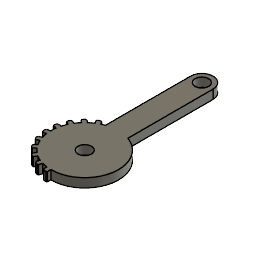
Record 11 3rd part (Autodesk Fusion 360 design; units mm, degrees)
part number: 2026-03-10-15-59-10-716
Autodesk Fusion 360 part; units mm, degrees
sketch "Sketch1" plane through (0, 0, 0) normal (0, 1, 0) x (1, 0, 0)
  circle A0 centre (0.0008, 24.9355) radius 3
  line L0 (2.5556, 32.9383) -> (-2.4444, 32.9383)
  line L1 (2.5556, 20.6375) -> (2.5556, -15.7025)
  line L2 (8, 25) -> (8, -20)
  circle A1 centre (0, -20) radius 3
  line L3 (-2.6799, 20.7149) -> (-2.6799, -15.7789)
  arc A2 (2.5556, 20.6375) -> (-2.6799, 20.7149) centre (0.0008, 24.9355) ccw
  arc A3 (-2.6799, -15.7789) -> (2.5556, -15.7025) centre (0, -20) ccw
  dimension "d1" = 6
  dimension "d2" = 10
  dimension "d4" = 5
  dimension "d5" = 36.34
  dimension "d6" = 45
  dimension "d7" = 6
  constraint concentric A0 A2
  constraint perpendicular L0 L1
  constraint vertical L2
  constraint concentric A1 A3
  constraint vertical L3
  constraint vertical L1
  measures "d1" diameter of A0
  measures "d2" diameter of A2
  measures "d4" distance of L0.start L0.end
  measures "d5" distance of L1.start L1.end
  measures "d6" distance of L2.start L2.end
  measures "d7" diameter of A1
sketch "Sketch2" plane through (0, 0, 0) normal (0, 1, 0) x (1, 0, 0)
  circle A0 centre (160, 0) radius 3
  line L0 (165.3043, -12.1067) -> (165.3043, 17.8933)
  line L1 (165.3043, -12.1067) -> (144.0787, -27.9224)
  line L2 (144.0787, -27.9224) -> (124.0787, -27.9224)
  line L3 (124.0787, -27.9224) -> (105.4535, -9.1138)
  line L4 (105.4535, -9.1138) -> (98.3535, -9.1138)
  line L5 (98.3535, -9.1138) -> (98.3535, 10.8862)
  line L6 (98.3535, 10.8862) -> (112.5535, 10.8862)
  line L7 (112.5535, 10.8862) -> (128, 34)
  line L8 (128, 34) -> (153, 34)
  line L9 (153, 34) -> (165.3043, 17.8933)
  circle A1 centre (144.0787, -15.0238) radius 3
  circle A2 centre (124.0787, -15.0238) radius 3
  line L10 (112.4283, -2.9974) -> (127.553, -3)
  line L11 (127.2855, 2.988) -> (112.556, 3)
  arc A3 (127.553, -3) -> (127.2855, 2.988) centre (127.5535, 0) ccw
  arc A4 (112.556, 3) -> (112.6778, -2.9974) centre (112.5535, 0) ccw
  circle A5 centre (128, 28) radius 2
  circle A6 centre (153, 28) radius 2
  dimension "d10" = 6
  dimension "d11" = 30
  dimension "d12" = 26.47
  dimension "d13" = 20
  dimension "d14" = 26.47
  dimension "d15" = 7.1
  dimension "d16" = 20
  dimension "d17" = 14.2
  dimension "d18" = 27.8
  dimension "d19" = 25
  dimension "d21" = 6
  dimension "d22" = 6
  dimension "d23" = 6
  dimension "d24" = 15
  dimension "d25" = 6
  dimension "d26" = 4
  dimension "d27" = 4
  constraint vertical L0
  constraint horizontal L2
  constraint horizontal L4
  constraint perpendicular L4 L5
  constraint perpendicular L5 L6
  constraint horizontal L8
  constraint coincident L10.start A4
  constraint tangent L10 A3
  constraint tangent L11 A4
  constraint coincident L10 A4.end
  measures "d10" diameter of A0
  measures "d11" distance of L0.start L0.end
  measures "d12" distance of L0.start L1.end
  measures "d13" distance of L1.end L2.end
  measures "d14" distance of L2.end L3.end
  measures "d15" distance of L3.end L4.end
  measures "d16" distance of L4.end L5.end
  measures "d17" distance of L5.end L6.end
  measures "d18" distance of L6.end L7.end
  measures "d19" distance of L7.end L8.end
  measures "d21" diameter of A1
  measures "d22" diameter of A2
  measures "d23" diameter of A4
  measures "d24" distance of A4.centre A3.centre
  measures "d25" diameter of A3
  measures "d26" diameter of A5
  measures "d27" diameter of A6
sketch "Sketch3" plane through (0, 0, 0) normal (0, 1, 0) x (1, 0, 0)
sketch "Sketch4" plane through (0, 0, 0) normal (0, 1, 0) x (1, 0, 0)
sketch "Sketch5" plane through (0, 0, 0) normal (0, 1, 0) x (1, 0, 0)
  circle A0 centre (0, -75) radius 3
  circle A1 centre (-0.0243, -126.973) radius 3
  line L0 (-20, -70) -> (-20, -141.97)
  line L1 (-5, -75) -> (-5, -112.8223)
  line L2 (5, -75) -> (5, -112.8395)
  arc A2 (5, -75) -> (-5, -75) centre (0, -75) ccw
  line L3 (-0.05, -141.973) -> (-0.05, -143.513)
  line L4 (-0.05, -143.513) -> (-0.4621, -143.739)
  line L5 (-0.4621, -143.739) -> (-1.4621, -143.739)
  line L6 (-1.4621, -143.739) -> (-1.9628, -143.2357)
  line L7 (-1.9628, -143.2357) -> (-1.9628, -141.8472)
  line L8 (-0.05, -145.0973) -> (-0.05, -123.9731)
  line L9 (-8.7204, -112.6318) -> (-7.8791, -112.0912)
  line L10 (-8.9448, -113.0448) -> (-8.7204, -112.6318)
  line L11 (-8.1122, -114.3403) -> (-8.9448, -113.0448)
  line L12 (-7.1857, -112.2439) -> (-6.4351, -113.412)
  line L13 (-7.8791, -112.0912) -> (-7.1857, -112.2439)
  line L14 (-12.4085, -115.6627) -> (-11.7536, -114.907)
  line L15 (-12.5075, -116.1222) -> (-12.4085, -115.6627)
  line L16 (-11.3436, -117.1306) -> (-12.5075, -116.1222)
  line L17 (-11.0453, -114.8581) -> (-9.996, -115.7674)
  line L18 (-11.7536, -114.907) -> (-11.0453, -114.8581)
  line L19 (-15.0933, -119.6099) -> (-14.6779, -118.7003)
  line L20 (-15.0589, -120.0786) -> (-15.0933, -119.6099)
  line L21 (-13.658, -120.7184) -> (-15.0589, -120.0786)
  line L22 (-14.012, -118.4539) -> (-12.749, -119.0307)
  line L23 (-14.6779, -118.7003) -> (-14.012, -118.4539)
  line L24 (-16.5573, -124.1536) -> (-16.415, -123.1638)
  line L25 (-16.3922, -124.5936) -> (-16.5573, -124.1536)
  line L26 (-14.8679, -124.8128) -> (-16.3922, -124.5936)
  line L27 (-15.8455, -122.7398) -> (-14.4712, -122.9374)
  line L28 (-16.415, -123.1638) -> (-15.8455, -122.7398)
  line L29 (-16.682, -128.9257) -> (-16.8243, -127.9359)
  line L30 (-16.3995, -129.3014) -> (-16.682, -128.9257)
  line L31 (-14.8752, -129.0822) -> (-16.3995, -129.3014)
  line L32 (-16.3973, -127.3686) -> (-15.023, -127.171)
  line L33 (-16.8243, -127.9359) -> (-16.3973, -127.3686)
  line L34 (-15.4571, -133.5396) -> (-15.8725, -132.63)
  line L35 (-15.0802, -133.8205) -> (-15.4571, -133.5396)
  line L36 (-13.6794, -133.1808) -> (-15.0802, -133.8205)
  line L37 (-15.6226, -131.9654) -> (-14.3596, -131.3886)
  line L38 (-15.8725, -132.63) -> (-15.6226, -131.9654)
  line L39 (-12.9819, -137.6215) -> (-13.6367, -136.8658)
  line L40 (-12.5412, -137.7849) -> (-12.9819, -137.6215)
  line L41 (-11.3773, -136.7764) -> (-12.5412, -137.7849)
  line L42 (-13.5843, -136.1577) -> (-12.5349, -135.2485)
  line L43 (-13.6367, -136.8658) -> (-13.5843, -136.1577)
  line L44 (-9.457, -140.8408) -> (-10.2982, -140.3002)
  line L45 (-8.9881, -140.8734) -> (-9.457, -140.8408)
  line L46 (-8.1555, -139.5779) -> (-8.9881, -140.8734)
  line L47 (-10.4473, -139.606) -> (-9.6967, -138.4379)
  line L48 (-10.2982, -140.3002) -> (-10.4473, -139.606)
  line L49 (-5.1679, -142.9365) -> (-6.1274, -142.6548)
  line L50 (-4.7088, -142.8357) -> (-5.1679, -142.9365)
  line L51 (-4.2749, -141.3581) -> (-4.7088, -142.8357)
  line L52 (-6.466, -142.0308) -> (-6.0748, -140.6985)
  line L53 (-6.1274, -142.6548) -> (-6.466, -142.0308)
  arc A3 (-5, -112.8223) -> (-6.4351, -113.412) centre (-0.0243, -126.973) ccw
  arc A4 (-8.1122, -114.3403) -> (-9.996, -115.7674) centre (-0.0243, -126.973) ccw
  arc A5 (-11.3436, -117.1306) -> (-12.749, -119.0307) centre (-0.0243, -126.973) ccw
  arc A6 (-13.658, -120.7184) -> (-14.4712, -122.9374) centre (-0.0243, -126.973) ccw
  arc A7 (-14.8679, -124.8128) -> (-15.023, -127.171) centre (-0.0243, -126.973) ccw
  arc A8 (-14.8752, -129.0822) -> (-14.3596, -131.3886) centre (-0.0243, -126.973) ccw
  arc A9 (-13.6794, -133.1808) -> (-12.5349, -135.2485) centre (-0.0243, -126.973) ccw
  arc A10 (-11.3773, -136.7764) -> (-9.6967, -138.4379) centre (-0.0243, -126.973) ccw
  arc A11 (-8.1555, -139.5779) -> (-6.0748, -140.6985) centre (-0.0243, -126.973) ccw
  arc A12 (-4.2749, -141.3581) -> (-1.9628, -141.8472) centre (-0.0243, -126.973) ccw
  arc A13 (-0.05, -141.973) -> (5, -112.8395) centre (-0.0243, -126.973) ccw
  dimension "d30" = 6
  dimension "d31" = 10
  dimension "d32" = 6
  dimension "d33" = 30
  dimension "d34" = 71.97
  dimension "d35" = 1.54
  dimension "d36" = 0.47
  dimension "d37" = 1
  dimension "d38" = 0.71
  dimension "d40" = 360
  constraint concentric A0 A2
  constraint concentric A1 A4
  constraint vertical L0
  constraint vertical L1
  constraint tangent L2 A2
  constraint parallel L1 L2
  constraint vertical L3
  constraint horizontal L5
  constraint vertical L7
  constraint vertical L8
  constraint coincident A1 L8.end
  constraint concentric A3 A4
  constraint concentric A4 A5
  constraint concentric A5 A6
  constraint concentric A6 A7
  constraint concentric A7 A8
  constraint concentric A8 A9
  constraint concentric A9 A10
  constraint concentric A10 A11
  constraint concentric A11 A12
  constraint concentric A12 A13
  measures "d30" diameter of A0
  measures "d31" diameter of A2
  measures "d32" diameter of A1
  measures "d33" diameter of A3
  measures "d34" distance of L0.start L0.end
  measures "d35" distance of L3.start L3.end
  measures "d36" distance of L3.end L4.end
  measures "d37" distance of L4.end L5.end
  measures "d38" distance of L5.end L6.end
extrude "Extrude3" add sketch "Sketch5" along normal blind 4
sketch "Sketch6" plane through (0, 0, 0) normal (0, 1, 0) x (1, 0, 0)
  circle A0 centre (135, -70) radius 3
  circle A1 centre (135, -95) radius 3
  line L0 (129.0014, -94.8707) -> (129, -70.0003)
  line L1 (141, -95) -> (141, -70)
  arc A2 (141, -70) -> (129, -70.0003) centre (135, -70) ccw
  line L2 (134.9353, -100.9997) -> (150.363, -126.7288)
  line L3 (138.9186, -99.5437) -> (196.6373, -196.6907)
  arc A3 (129.0014, -94.8707) -> (134.9353, -100.9997) centre (135, -95) ccw
  arc A4 (138.9186, -99.5437) -> (141, -95) centre (135, -95) ccw
  line L4 (196.6373, -196.6907) -> (189.4976, -203.5489)
  line L5 (189.4976, -203.5489) -> (182.5189, -204.0946)
  line L6 (150.363, -126.7288) -> (142.6345, -134.4043)
  line L7 (179.3777, -201.8435) -> (142.738, -137.5509)
  arc A5 (179.3777, -201.8435) -> (182.5189, -204.0946) centre (182.2851, -201.1037) ccw
  arc A6 (142.6345, -134.4043) -> (142.738, -137.5509) centre (145.2387, -135.8936) ccw
  dimension "d43" = 6
  dimension "d44" = 12
  dimension "d45" = 25
  dimension "d46" = 6
  dimension "d47" = 12
  dimension "d48" = 30
  dimension "d50" = 113
  dimension "d52" = 9.9
  dimension "d53" = 7
  dimension "d62" = 6
  dimension "d63" = 74
  dimension "d64" = 6
  constraint concentric A0 A2
  constraint concentric A1 A3
  constraint tangent L0 A2
  constraint tangent L1 A2
  constraint concentric A3 A4
  constraint tangent L5 A5
  constraint coincident L5 A5.end
  measures "d43" diameter of A0
  measures "d44" diameter of A2
  measures "d45" distance of A0.centre A1.centre
  measures "d46" diameter of A1
  measures "d47" diameter of A3
  measures "d48" distance of L2.start L2.end
  measures "d50" distance of L3.start L3.end
  measures "d52" distance of L3.end L4.end
  measures "d53" distance of L4.end L5.end
  measures "d62" diameter of A5
  measures "d63" distance of L7.start L7.end
  measures "d64" diameter of A6
